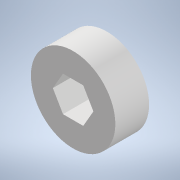
# Autodesk Inventor part: Rodamiento_Ejes
Saved by Autodesk Inventor 2022 (Build 260153000, 153)
## iProperties
Created: 2022-02-21
Part Number: Rodamiento_Ejes
Material: Generic
Document SubType Name: Modeling
Designer: katha
Density: 1 g/cm^3
Appearance: Default
Author: katha
Autodesk Inventor part; units mm, degrees
ref_plane "YZ Plane" through (0, 0, 0) normal (1, 0, 0) x (0, 1, 0)
ref_plane "XZ Plane" through (0, 0, 0) normal (0, 1, 0) x (-1, 0, 0)
ref_plane "XY Plane" through (0, 0, 0) normal (0, 0, 1) x (1, 0, 0)
sketch "Sketch1" plane through (0, 0, 0) normal (0, 0, 1) x (1, 0, 0)
  line L0 (-1.6732, 2.8981) -> (1.6732, 2.8981) projected
  line L1 (-3.3464, 0) -> (-1.6732, 2.8981) projected
  line L2 (-1.6732, -2.8981) -> (-3.3464, 0) projected
  line L3 (1.6732, -2.8981) -> (-1.6732, -2.8981) projected
  line L4 (3.3464, 0) -> (1.6732, -2.8981) projected
  line L5 (1.6732, 2.8981) -> (3.3464, 0) projected
  circle A0 centre (0, 0) radius 7.5
  constraints: 1 centre point
extrude "Extrusion1" add sketch "Sketch1" against normal blind 6
sketch "Sketch2" plane through (0, 0, 0) normal (0, 0, 1) x (1, 0, 0)
  circle A0 centre (0, 0) radius 7.5 projected
  line L0 (0, 0) -> (-3.1, 0) construction
  line L1 (0, 0) -> (-1.55, -2.6847) construction
  line L2 (0, 0) -> (1.55, -2.6847) construction
  line L3 (0, 0) -> (3.1, 0) construction
  line L4 (0, 0) -> (1.55, 2.6847) construction
  line L5 (0, 0) -> (-1.55, 2.6847) construction
  line L6 (1.55, 2.6847) -> (-1.55, 2.6847) construction
  line L7 (1.6732, 2.8981) -> (-1.6732, 2.8981) projected
  line L8 (-1.55, 2.6847) -> (-3.1, 0) construction
  line L9 (1.55, -2.6847) -> (-1.55, -2.6847) construction
  line L10 (-1.6732, -2.8981) -> (1.6732, -2.8981) projected
  line L11 (-1.55, -2.6847) -> (-3.1, 0) construction
  line L12 (1.55, -2.6847) -> (3.1, 0) construction
  line L13 (3.1, 0) -> (1.55, 2.6847) construction
  line L14 (3.3464, 0) -> (1.6732, 2.8981) projected
  line L15 (-1.7809, 3.0847) -> (1.7809, 3.0847)
  line L16 (1.7809, 3.0847) -> (3.5619, 0)
  line L17 (3.5619, 0) -> (1.7809, -3.0847)
  line L18 (1.7809, -3.0847) -> (-1.7809, -3.0847)
  line L19 (-1.7809, -3.0847) -> (-3.5619, 0)
  line L20 (-3.5619, 0) -> (-1.7809, 3.0847)
  point P0 (0, 0)
  dimension "d4" = 3.1
  dimension "d7" = 360
  dimension "d9" = 0.4
  constraints: 36 end point, 3 parallel, 2 coincident, 1 horizontal, 22 other
  measures "d4" distance of L0.start L0.end
  measures "d9" distance between parallel lines of L6 L15
extrude "Extrusion2" cut sketch "Sketch2" against normal blind 10 contours L15 L16 L17 L18 L19 L20
body "Solid1"
